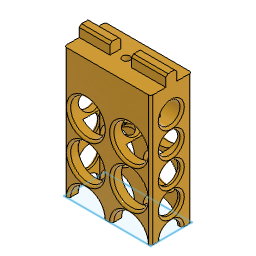
foot v2 (Autodesk Fusion 360 design; units mm, degrees)
Autodesk Fusion 360 part; units mm, degrees
sketch "Skizze1" plane through (0, 0, 0) normal (0, 0, 1) x (1, 0, 0)
  line L0 (10, 25) -> (50, 25)
  line L1 (50, 25) -> (50, 6)
  line L2 (50, 6) -> (10, 6)
  line L3 (10, 6) -> (10, 25)
  dimension "d1" = 40
  dimension "d2" = 19
  constraint horizontal L0
  constraint vertical L1
  constraint horizontal L2
  constraint vertical L3
  measures "d1" distance of L0.start L0.end
  measures "d2" distance of L0.start L2.end
extrude "Extrusion1" add sketch "Skizze1" along normal blind 60
sketch "Skizze2" plane through (0, 0, 60) normal (0, 0, 1) x (-1, 0, 0)
  line L0 (-10, -6) -> (-50, -6)
  line L1 (-50, -6) -> (-50, -25)
  line L2 (-50, -25) -> (-10, -25)
  line L3 (-10, -25) -> (-10, -6)
  line L4 (-10, -15.5) -> (-50, -15.5) construction
  line L5 (-10, -13) -> (-50, -13)
  line L6 (-10, -18) -> (-50, -18)
  constraint midpoint L3 L4.start
  constraint midpoint L1 L4.end
extrude "Extrusion2" add sketch "Skizze2" along normal blind 5 contours L1 L3 L5 L6
chamfer "Fase1" distance 1 angle 45 1 edges at (30, 13, 65)
chamfer "Fase2" distance 1 angle 45 1 edges at (30, 18, 65)
sketch "Skizze3" plane through (0, 0, 65) normal (0, 0, 1) x (-1, 0, 0)
  line L0 (-50, -17) -> (-10, -17)
  line L1 (-10, -17) -> (-10, -14)
  line L2 (-10, -14) -> (-50, -14)
  line L3 (-50, -14) -> (-50, -17)
  line L4 (-10, -17) -> (-50, -14) construction
  line L5 (-24.1578, -17.9999) -> (-34.1578, -17.9999)
  line L6 (-34.1578, -17.9999) -> (-34.1578, -12.9999)
  line L7 (-34.1578, -12.9999) -> (-24.1578, -12.9999)
  line L8 (-24.1578, -12.9999) -> (-24.1578, -17.9999)
  dimension "d11" = 10
  dimension "d12" = 5
  constraint coincident L0.end L1.start
  constraint coincident L2.end L3.start
  constraint horizontal L5
  constraint vertical L6
  constraint horizontal L7
  constraint vertical L8
  measures "d11" distance of L5.start L5.end
  measures "d12" distance of L5.start L7.end
extrude "Extrusion3" cut sketch "Skizze3" against normal blind 5 contours L0 L2 L6 L8 | L0 L5 L6 L8 | L2 L6 L7 L8
delete_face "Fläche löschen1" 1 faces at (27.4912, 17.9999, 62.6667)
sketch "Skizze4" plane through (0, 0, 60) normal (0, 0, 1) x (-1, 0, 0)
  line L0 (-24.1578, -18) -> (-24.1578, -13)
  line L1 (-24.1578, -13) -> (-10, -13)
  line L2 (-10, -13) -> (-10, -6)
  line L3 (-10, -6) -> (-50, -6)
  line L4 (-50, -6) -> (-50, -13)
  line L5 (-50, -13) -> (-34.1578, -13)
  line L6 (-34.1578, -13) -> (-34.1578, -18)
  line L7 (-34.1578, -18) -> (-50, -18)
  line L8 (-50, -18) -> (-50, -25)
  line L9 (-50, -25) -> (-10, -25)
  line L10 (-10, -25) -> (-10, -18)
  line L11 (-10, -18) -> (-24.1578, -18)
  line L12 (-24.1578, -18) -> (-34.1578, -13) construction
  circle A0 centre (-29.1578, -15.5) radius 1.75
  dimension "d15" = 3.5
  constraint coincident L0.start L11.end
  constraint coincident L5.end L6.start
  constraint midpoint L12 A0.centre
  measures "d15" diameter of A0
extrude "Extrusion4" cut sketch "Skizze4" against normal blind 71 contours A0
sketch "Skizze5" plane through (0, 0, 60) normal (0, 0, 1) x (-1, 0, 0)
  circle A0 centre (-29.1578, -15.5) radius 1.75
  line L0 (-24.1578, -18) -> (-24.1578, -13)
  line L1 (-24.1578, -13) -> (-10, -13)
  line L2 (-10, -13) -> (-10, -6)
  line L3 (-10, -6) -> (-50, -6)
  line L4 (-50, -6) -> (-50, -13)
  line L5 (-50, -13) -> (-34.1578, -13)
  line L6 (-34.1578, -13) -> (-34.1578, -18)
  line L7 (-34.1578, -18) -> (-50, -18)
  line L8 (-50, -18) -> (-50, -25)
  line L9 (-50, -25) -> (-10, -25)
  line L10 (-10, -25) -> (-10, -18)
  line L11 (-10, -18) -> (-24.1578, -18)
sketch "Skizze7" plane through (0, 0, 0) normal (0, 0, -1) x (1, 0, 0)
  circle A0 centre (29.1578, -15.5) radius 1.75
  line L0 (50, -6) -> (10, -6)
  line L1 (10, -6) -> (10, -25)
  line L2 (10, -25) -> (50, -25)
  line L3 (50, -25) -> (50, -6)
  circle A1 centre (29.1578, -15.5) radius 3
  dimension "d19" = 6
  constraint concentric A0 A1
  measures "d19" diameter of A1
extrude "Extrusion5" cut sketch "Skizze7" against normal blind 55 contours A1
sketch "Skizze6" plane through (0, 0, 0) normal (0, 0, 1) x (1, 0, 0)
sketch "Skizze8" plane through (50, 0, 0) normal (1, 0, 0) x (0, 1, 0)
  line L0 (18, 64) -> (17, 65)
  line L1 (17, 65) -> (14, 65)
  line L2 (14, 65) -> (13, 64)
  line L3 (13, 64) -> (13, 60)
  line L4 (13, 60) -> (6, 60)
  line L5 (6, 60) -> (6, 0)
  line L6 (6, 0) -> (25, 0)
  line L7 (25, 0) -> (25, 60)
  line L8 (25, 60) -> (18, 60)
  line L9 (18, 60) -> (18, 64)
  line L10 (15.5, 0) -> (15.5, 65) construction
  circle A0 centre (15.5, 0) radius 5
  circle A1 centre (15.5, 12) radius 5
  circle A2 centre (15.5, 24) radius 5
  circle A3 centre (15.5, 36) radius 5
  circle A4 centre (15.5, 48) radius 5
  dimension "d22" = 10
  dimension "d23" = 10
  dimension "d24" = 10
  dimension "d25" = 10
  dimension "d26" = 10
  constraint midpoint L6 L10.start
  constraint midpoint L1 L10.end
  constraint coincident L10.start A0.centre
  measures "d22" diameter of A0
  measures "d23" diameter of A1
  measures "d24" diameter of A2
  measures "d25" diameter of A3
  measures "d26" diameter of A4
extrude "Extrusion6" cut sketch "Skizze8" against normal blind 47 contours L6 A0 | A1 | A2 | A3 | A4 picked at (16.8771, 0.9389)
sketch "Skizze9" plane through (0, 6, 0) normal (0, -1, 0) x (1, 0, 0)
  line L0 (10, 0) -> (50, 0)
  line L1 (50, 0) -> (50, 60)
  line L2 (50, 60) -> (10, 60)
  line L3 (10, 60) -> (10, 0)
  line L4 (30, 0) -> (30, 60) construction
  line L5 (20, 0) -> (20, 60) construction
  line L6 (40.1834, 0) -> (40.1834, 60) construction
  circle A0 centre (20, 0) radius 8
  circle A1 centre (20, 18) radius 8
  circle A2 centre (20, 36) radius 8
  circle A3 centre (40, 36) radius 8
  circle A4 centre (40, 18) radius 8
  circle A5 centre (40, 0) radius 8
  dimension "d29" = 16
  dimension "d30" = 16
  dimension "d31" = 16
  dimension "d32" = 16
  dimension "d33" = 16
  dimension "d34" = 16
  constraint midpoint L0 L4.start
  constraint midpoint L2 L4.end
  constraint coincident L0 L5.start
  constraint coincident L2 L5.end
  constraint perpendicular L2 L5
  constraint coincident L0 L6.start
  constraint coincident L2 L6.end
  constraint perpendicular L2 L6
  constraint coincident L5.start A0.centre
  measures "d29" diameter of A0
  measures "d30" diameter of A1
  measures "d31" diameter of A2
  measures "d32" diameter of A5
  measures "d33" diameter of A4
  measures "d34" diameter of A3
extrude "Extrusion7" cut sketch "Skizze9" against normal blind 52 contours L0 A5 | L0 A0 | A1 | A2 | A3 | A4 picked at (42.4376, 3.0567) picked at (21.6924, 2.4823)
sketch "Skizze10" plane through (0, 0, 0) normal (0, 0, 1) x (1, 0, 0)
  line L0 (50, 6) -> (10, 25) construction
  line L1 (12, 10.5) -> (48, 10.5)
  line L2 (48, 10.5) -> (48, 20.5)
  line L3 (48, 20.5) -> (12, 20.5)
  line L4 (12, 20.5) -> (12, 10.5)
  constraint horizontal L1
  constraint vertical L2
  constraint horizontal L3
  constraint vertical L4
extrude "Extrusion8" cut sketch "Skizze10" along normal blind 30.5
fillet "Abrundung1" radius 1 1 edges at (50, 6, 30)
fillet "Abrundung2" radius 1 2 edges at (10, 6, 30) (50, 25, 30)
fillet "Abrundung3" radius 1 1 edges at (10, 25, 30)
fillet "Abrundung4" radius 1 1 edges at (50, 10.8384, 49.8081)
fillet "Abrundung5" radius 1 3 edges at (50, 10.8384, 37.8081) (50, 10.8384, 25.8081) (50, 10.8384, 13.8081)
fillet "Abrundung6" radius 1 4 edges at (32.5414, 25, 33.1071) (12.5414, 25, 33.1071) (12.5414, 25, 15.1071) (32.5414, 25, 15.1071)
fillet "Abrundung7" radius 1 1 edges at (50, 15.5, 5)
fillet "Abrundung8" radius 1 1 edges at (20, 25, 8)
fillet "Abrundung9" radius 1 tangency weight 1.14648 1 edges at (40, 25, 8)
fillet "Abrundung10" radius 1 5 edges at (10, 15.5, 5) (10, 10.8384, 10.1919) (10, 10.8384, 22.1919) (10, 10.8384, 34.1919) (10, 10.8384, 46.1919)
fillet "Abrundung11" radius 1 6 edges at (12.5414, 6, 38.8929) (32.5414, 6, 38.8929) (12.5414, 6, 20.8929) (32.5414, 6, 20.8929) (40, 6, 8) (20, 6, 8)
